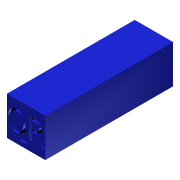
# Autodesk Inventor part: Container 2 2 5 QR color 4
Saved by Autodesk Inventor 2015 (Build 190159000, 159)
## iProperties
Created: 2015-03-07
Part Number: Container 2 2 5 QR color 4
Material: Generic
Document SubType Name: Modeling
Designer: Vukica
Density: 1 g/cm^3
Appearance: Red
Author: Vukica
Autodesk Inventor part; units mm, degrees
ref_plane "YZ Plane" through (0, 0, 0) normal (1, 0, 0) x (0, 1, 0)
ref_plane "XZ Plane" through (0, 0, 0) normal (0, 1, 0) x (-1, 0, 0)
ref_plane "XY Plane" through (0, 0, 0) normal (0, 0, 1) x (1, 0, 0)
sketch "Sketch1" plane through (0, 0, 0) normal (0, 0, 1) x (1, 0, 0)
  line L0 (0, 0) -> (38.1, 0)
  line L1 (38.1, 0) -> (38.1, 38.1)
  line L2 (38.1, 38.1) -> (0, 38.1)
  line L3 (0, 38.1) -> (0, 0)
  dimension "d0" = 38.1
  dimension "d1" = 38.1
  constraints: 8 end point, 2 parallel, 1 horizontal, 1 perpendicular
  measures "d0" distance of L1.end L2.end
  measures "d1" distance of L2.end L0.start
extrude "Extrusion1" add sketch "Sketch1" along normal blind 127
sketch "Sketch2" plane through (0, 0, 127) normal (0, 0, 1) x (1, 0, 0)
  line L0 (0.2863, 30.2826) -> (46.6814, 30.2826) construction
  line L1 (46.6814, 30.2826) -> (46.6814, -2.3422) construction
  line L2 (46.6814, -2.3422) -> (0.2863, -2.3422) construction
  line L3 (0.2863, -2.3422) -> (0.2863, 30.2826) construction
  spline S0 degree 2 poles (19.2231, 4.5615) (18.4821, 4.3804) (16.8683, 4.1828) (16.0614, 4.1828) knots 0 0 0 1 2 2 2
  spline S1 degree 2 poles (16.0614, 4.1828) (13.7726, 4.1828) (10.9238, 6.7352) (10.7921, 9.1064) knots 0 0 0 1 2 2 2
  spline S2 degree 2 poles (10.7921, 9.1064) (10.6109, 9.1064) (10.2981, 9.1064) (10.1663, 9.1064) knots 0 0 0 1 2 2 2
  spline S3 degree 2 poles (10.1663, 9.1064) (8.108, 9.1064) (4.7982, 10.506) (3.6126, 11.8728) knots 0 0 0 1 2 2 2
  spline S4 degree 2 poles (3.6126, 11.8728) (2.4434, 13.2231) (1.1919, 17.1751) (1.1919, 19.678) knots 0 0 0 1 2 2 2
  spline S5 degree 2 poles (1.1919, 19.678) (1.1919, 22.2469) (2.4599, 26.133) (3.629, 27.5162) knots 0 0 0 1 2 2 2
  spline S6 degree 2 poles (3.629, 27.5162) (4.8146, 28.883) (8.1245, 30.2826) (10.1663, 30.2826) knots 0 0 0 1 2 2 2
  spline S7 degree 2 poles (10.1663, 30.2826) (12.2412, 30.2826) (15.5674, 28.8336) (16.7201, 27.5162) knots 0 0 0 1 2 2 2
  spline S8 degree 2 poles (16.7201, 27.5162) (17.8728, 26.1824) (19.1572, 22.2139) (19.1572, 19.678) knots 0 0 0 1 2 2 2
  spline S9 degree 2 poles (19.1572, 19.678) (19.1572, 15.726) (16.0779, 10.5884) (13.3938, 9.6827) knots 0 0 0 1 2 2 2
  spline S10 degree 2 poles (13.3938, 9.6827) (13.4597, 8.9252) (13.8549, 7.7067) (14.1678, 7.3609) knots 0 0 0 1 2 2 2
  spline S11 degree 2 poles (14.1678, 7.3609) (14.5465, 6.9328) (15.5839, 6.5376) (16.5061, 6.5376) knots 0 0 0 1 2 2 2
  spline S12 degree 2 poles (16.5061, 6.5376) (17.0495, 6.5376) (18.5315, 6.8834) (18.8608, 7.0151) knots 0 0 0 1 2 2 2
  line L4 (18.8608, 7.0151) -> (19.2231, 7.0151)
  line L5 (19.2231, 7.0151) -> (19.2231, 4.5615)
  spline S13 degree 2 poles (16.3414, 19.678) (16.3414, 21.7035) (15.4686, 24.8157) (14.6782, 25.8366) knots 0 0 0 1 2 2 2
  spline S14 degree 2 poles (14.6782, 25.8366) (13.8714, 26.8905) (11.599, 27.9444) (10.1828, 27.9444) knots 0 0 0 1 2 2 2
  spline S15 degree 2 poles (10.1828, 27.9444) (8.7173, 27.9444) (6.5107, 26.9234) (5.6709, 25.8366) knots 0 0 0 1 2 2 2
  spline S16 degree 2 poles (5.6709, 25.8366) (4.864, 24.7992) (4.0078, 21.6541) (4.0078, 19.678) knots 0 0 0 1 2 2 2
  spline S17 degree 2 poles (4.0078, 19.678) (4.0078, 15.6766) (7.367, 11.4117) (10.1828, 11.4117) knots 0 0 0 1 2 2 2
  spline S18 degree 2 poles (10.1828, 11.4117) (12.9986, 11.4117) (16.3414, 15.6766) (16.3414, 19.678) knots 0 0 0 1 2 2 2
  line L6 (37.847, 9.5345) -> (34.3396, 9.5345)
  line L7 (34.3396, 9.5345) -> (27.9175, 17.6197)
  line L8 (27.9175, 17.6197) -> (24.8218, 17.6197)
  line L9 (24.8218, 17.6197) -> (24.8218, 9.5345)
  line L10 (24.8218, 9.5345) -> (22.1212, 9.5345)
  line L11 (22.1212, 9.5345) -> (22.1212, 29.8545)
  line L12 (22.1212, 29.8545) -> (27.3577, 29.8545)
  spline S19 degree 2 poles (27.3577, 29.8545) (29.1031, 29.8545) (31.4579, 29.4758) (32.5282, 28.7842) knots 0 0 0 1 2 2 2
  spline S20 degree 2 poles (32.5282, 28.7842) (33.5986, 28.0926) (34.8336, 25.9354) (34.8336, 24.3381) knots 0 0 0 1 2 2 2
  spline S21 degree 2 poles (34.8336, 24.3381) (34.8336, 22.1151) (32.5612, 19.1017) (30.6181, 18.3772) knots 0 0 0 1 2 2 2
  line L13 (30.6181, 18.3772) -> (37.847, 9.5345)
  spline S22 degree 2 poles (32.0178, 24.1241) (32.0178, 25.0133) (31.392, 26.38) (30.7333, 26.8246) knots 0 0 0 1 2 2 2
  spline S23 degree 2 poles (30.7333, 26.8246) (30.157, 27.2034) (28.6256, 27.5162) (27.5059, 27.5162) knots 0 0 0 1 2 2 2
  line L14 (27.5059, 27.5162) -> (24.8218, 27.5162)
  line L15 (24.8218, 27.5162) -> (24.8218, 19.8756)
  line L16 (24.8218, 19.8756) -> (27.193, 19.8756)
  spline S24 degree 2 poles (27.193, 19.8756) (28.3621, 19.8756) (30.2229, 20.2873) (30.8651, 20.9295) knots 0 0 0 1 2 2 2
  spline S25 degree 2 poles (30.8651, 20.9295) (31.4579, 21.4894) (32.0178, 23.0702) (32.0178, 24.1241) knots 0 0 0 1 2 2 2
  point P0 (0, 0)
  constraints: 2 other
extrude "Extrusion2" cut sketch "Sketch2" against normal blind 2.54
body "Solid1"
